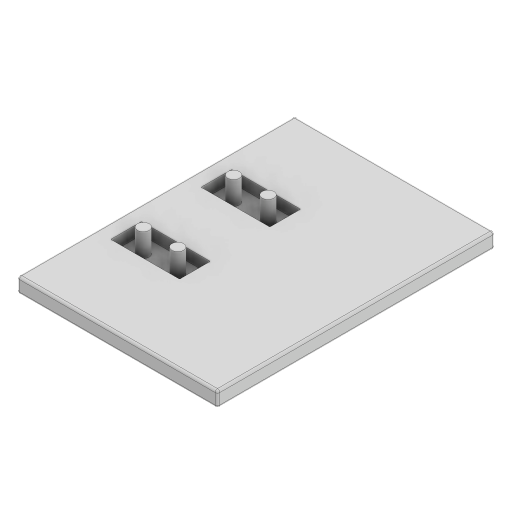
# Autodesk Inventor part: base2
Saved by Autodesk Inventor 2024 (Build 280153000, 153)
## iProperties
Created: 2024-04-22
Part Number: base2
Material: Generic
Document SubType Name: Modeling
Designer: alexz
Density: 1 g/cm^3
Appearance: Default
Author: alexz
Autodesk Inventor part; units mm, degrees
ref_plane "YZ Plane" through (0, 0, 0) normal (1, 0, 0) x (0, 1, 0)
ref_plane "XZ Plane" through (0, 0, 0) normal (0, 1, 0) x (-1, 0, 0)
ref_plane "XY Plane" through (0, 0, 0) normal (0, 0, 1) x (1, 0, 0)
sketch "Sketch1" plane through (0, 0, 0) normal (0, 1, 0) x (-1, 0, 0)
  line L0 (0, 0) -> (260, 0)
  line L1 (260, 0) -> (260, -360)
  line L2 (260, -360) -> (0, -360)
  line L3 (0, -360) -> (0, 0)
  line L4 (240, -101.4) -> (150.6, -101.4)
  line L5 (150.6, -101.4) -> (150.6, -141.4)
  line L6 (150.6, -141.4) -> (240, -141.4)
  line L7 (240, -141.4) -> (240, -101.4)
  line L8 (240, -218.6) -> (150.6, -218.6)
  line L9 (150.6, -218.6) -> (150.6, -258.6)
  line L10 (150.6, -258.6) -> (240, -258.6)
  line L11 (240, -258.6) -> (240, -218.6)
  circle A0 centre (217.65, -121.4) radius 7.5
  circle A1 centre (172.95, -121.4) radius 7.5
  circle A2 centre (217.65, -238.6) radius 7.5
  circle A3 centre (172.95, -238.6) radius 7.5
  point P0 (240, -121.4)
  point P1 (150.6, -238.6)
  point P2 (240, -238.6)
  dimension "d0" = 260
  dimension "d1" = 360
  dimension "d2" = 89.4
  dimension "d3" = 40
  dimension "d4" = 89.4
  dimension "d5" = 40
  dimension "d8" = 15
  dimension "d9" = 15
  dimension "d11" = 22.35
  dimension "d12" = 15
  dimension "d13" = 15
  dimension "d14" = 22.35
  dimension "d15" = 22.35
  dimension "d16" = 22.35
  dimension "d17" = 20
  dimension "d61" = 117.2
  dimension "d62" = 101.4
  dimension "d63" = 101.4
  constraints: 24 end point, 5 parallel, 4 centre point, 4 horizontal alignment, 3 horizontal, 3 midpoint, 3 perpendicular, 1 vertical alignment
  measures "d0" distance of L1.end L2.end
  measures "d1" distance of L0.end L1.end
  measures "d2" distance of L6.end L5.end
  measures "d3" distance of L5.end L4.end
  measures "d4" distance of L10.end L9.end
  measures "d5" distance of L9.end L8.end
  measures "d8" diameter of A0
  measures "d9" diameter of A1
  measures "d11" distance from line of A1.centre L5
  measures "d12" diameter of A2
  measures "d13" diameter of A3
  measures "d14" distance from line of A0.centre L7
  measures "d15" distance from line of L11 A2.centre
  measures "d16" distance of A3.centre point (150.6, -238.6)
  measures "d17" distance between parallel lines of L1 L7
  measures "d61" distance of point (240, -238.6) point (240, -121.4)
  measures "d62" distance between parallel lines of L0 L4
  measures "d63" distance between parallel lines of L2 L10
extrude "Extrusion1" add sketch "Sketch1" along normal blind 20 contours L0 L1 L2 L3
extrude "Extrusion2" add sketch "Sketch1" along normal blind 5 contours L7 L6 L5 L4 | L11 L10 L9 L8
extrude "Extrusion3" add sketch "Sketch1" along normal blind 35 contours A0 | A1 | A2 | A3
sketch "Sketch2" plane through (0, 20, 0) normal (0, 1, 0) x (1, 0, 0)
  point P0 (0, 0)
sketch "Sketch4" plane through (0, 0, 0) normal (0, -1, 0) x (1, 0, 0)
  line L0 (-240, -335) -> (-240, -320) construction
  line L1 (-235, -335) -> (-235, -320)
  line L2 (-245, -320) -> (-245, -335)
  arc A0 (-245, -335) -> (-235, -335) centre (-240, -335) ccw
  arc A1 (-235, -320) -> (-245, -320) centre (-240, -320) ccw
  line L3 (-260, -360) -> (-260, 0) projected
  line L4 (0, -360) -> (-260, -360) projected
  line L5 (-240, -40) -> (-240, -25) construction
  line L6 (-235, -40) -> (-235, -25)
  line L7 (-245, -25) -> (-245, -40)
  arc A2 (-245, -40) -> (-235, -40) centre (-240, -40) ccw
  arc A3 (-235, -25) -> (-245, -25) centre (-240, -25) ccw
  line L8 (-20, -40) -> (-20, -25) construction
  line L9 (-15, -40) -> (-15, -25)
  line L10 (-25, -25) -> (-25, -40)
  arc A4 (-25, -40) -> (-15, -40) centre (-20, -40) ccw
  arc A5 (-15, -25) -> (-25, -25) centre (-20, -25) ccw
  line L11 (-20, -335) -> (-20, -320) construction
  line L12 (-15, -335) -> (-15, -320)
  line L13 (-25, -320) -> (-25, -335)
  arc A6 (-25, -335) -> (-15, -335) centre (-20, -335) ccw
  arc A7 (-15, -320) -> (-25, -320) centre (-20, -320) ccw
  line L14 (0, 0) -> (0, -360) projected
  line L15 (-260, 0) -> (0, 0) projected
  point P0 (-240, -327.5)
  point P1 (-240, -340)
  point P2 (-240, -32.5)
  point P3 (-240, -45)
  point P4 (-20, -32.5)
  point P5 (-20, -45)
  point P6 (-20, -327.5)
  point P7 (-20, -340)
  point P8 (-20, -20)
  point P9 (-240, -20)
  dimension "d39" = 15
  dimension "d40" = 10
  dimension "d41" = 20
  dimension "d42" = 20
  dimension "d43" = 15
  dimension "d44" = 10
  dimension "d45" = 15
  dimension "d46" = 10
  dimension "d47" = 15
  dimension "d48" = 10
  dimension "d49" = 20
  dimension "d50" = 20
  dimension "d51" = 20
  dimension "d52" = 20
  dimension "d53" = 20
  dimension "d54" = 20
  constraints: 32 end point, 22 point on circle, 16 tangent, 8 centre point, 4 midpoint, 4 parallel, 4 vertical
  measures "d39" distance of L0.start L0.end
  measures "d40" diameter of A1
  measures "d41" distance from line of L3 point (-240, -340)
  measures "d42" distance from line of L4 point (-240, -340)
  measures "d43" distance of L5.start L5.end
  measures "d44" diameter of A3
  measures "d45" distance of L8.start L8.end
  measures "d46" diameter of A5
  measures "d47" distance of L11.start L11.end
  measures "d48" diameter of A7
  measures "d49" distance from line of L14 point (-20, -340)
  measures "d50" distance from line of L4 point (-20, -340)
  measures "d51" distance from line of L15 point (-20, -20)
  measures "d52" distance from line of L14 point (-20, -20)
  measures "d53" distance from line of L3 point (-240, -20)
  measures "d54" distance from line of L15 point (-240, -20)
extrude "Extrusion5" add sketch "Sketch4" along normal blind 1 contours A0 L2 A1 L1 | A2 L7 A3 L6 | A4 L10 A5 L9 | A6 L13 A7 L12
fillet "Fillet1" radius 3 12 edges at (-260, 20, -180) (-130, 20, 0) (-260, 10, 0) (-130, 0, 0) (0, 10, 0) (0, 20, -180) (0, 0, -180) (-130, 0, -360) (-130, 20, -360) (0, 10, -360) (-260, 10, -360) (-260, 0, -180)
fillet "Fillet2" radius 1 8 edges at (-240, 12.5, -258.6) (-240, 12.5, -218.6) (-150.6, 12.5, -218.6) (-150.6, 12.5, -258.6) (-240, 12.5, -141.4) (-150.6, 12.5, -141.4) (-150.6, 12.5, -101.4) (-240, 12.5, -101.4)
body "Solid1"
